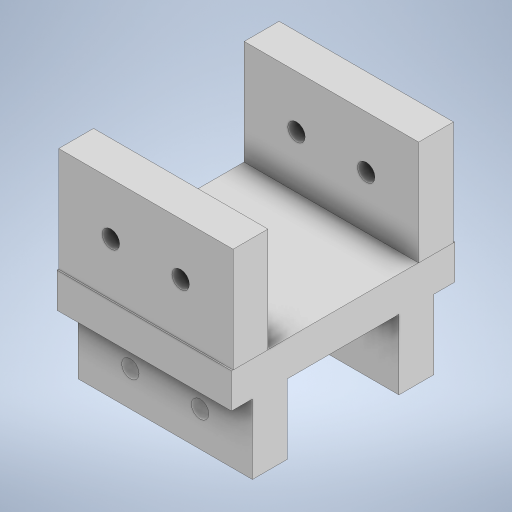
# Autodesk Inventor part: Tensile_test_bottom_adapter2
Saved by Autodesk Inventor 2024 (Build 280153000, 153)
## iProperties
Created: 2023-10-26
Part Number: Tensile_test_bottom_adapter2
Material: 일반
Document SubType Name: Modeling
Designer: jsw
Density: 1 g/cm^3
Appearance: 기본값
Author: jsw
Autodesk Inventor part; units mm, degrees
ref_plane "YZ Plane" through (0, 0, 0) normal (1, 0, 0) x (0, 1, 0)
ref_plane "XZ Plane" through (0, 0, 0) normal (0, 1, 0) x (-1, 0, 0)
ref_plane "XY Plane" through (0, 0, 0) normal (0, 0, 1) x (1, 0, 0)
sketch "스케치1" plane through (0, 0, 0) normal (0, 1, 0) x (-1, 0, 0)
  line L0 (-12.5, 16) -> (12.5, 16)
  line L1 (12.5, 16) -> (12.5, -16)
  line L2 (12.5, -16) -> (-12.5, -16)
  line L3 (-12.5, -16) -> (-12.5, 16)
  line L4 (-12.5, 16) -> (12.5, -16) construction
  line L5 (12.5, 16) -> (-12.5, -16) construction
  point P0 (0, 0)
  dimension "d0" = 25
  dimension "d1" = 32
  constraints: 12 end point, 2 midpoint, 2 parallel, 1 horizontal, 1 perpendicular
  measures "d0" distance of L1.end L2.end
  measures "d1" distance of L0.end L1.end
extrude "돌출1" add sketch "스케치1" along normal blind 5
sketch "스케치2" plane through (0, 5, 0) normal (0, 1, 0) x (1, 0, 0)
  line L0 (-12.4719, -15.8) -> (12.5281, -15.8)
  line L1 (12.5281, -15.8) -> (12.5281, -10.8)
  line L2 (12.5281, -10.8) -> (-12.4719, -10.8)
  line L3 (-12.4719, -10.8) -> (-12.4719, -15.8)
  line L4 (-12.5, 16) -> (-12.5, -16) projected
  line L5 (-12.5, 0) -> (12.5281, 0)
  line L6 (-12.4719, 15.8) -> (12.5281, 15.8)
  line L7 (12.5281, 15.8) -> (12.5281, 10.8)
  line L8 (12.5281, 10.8) -> (-12.4719, 10.8)
  line L9 (-12.4719, 10.8) -> (-12.4719, 15.8)
  line L10 (-12.5, -16) -> (-12.5, 16)
  point P0 (0, 0)
  dimension "d4" = 25
  dimension "d5" = 5
  dimension "d24" = 21.6
  constraints: 20 end point, 6 symmetric about line, 2 horizontal, 2 parallel, 1 midpoint, 1 perpendicular
  measures "d4" distance of L2.end L1.end
  measures "d5" distance of L1.end L0.end
  measures "d24" distance between parallel lines of L8 L2
extrude "돌출2" add sketch "스케치2" along normal blind 15
sketch "스케치3" plane through (12.5, 5, -15.8) normal (0, 0, -1) x (-1, 0, 0)
  circle A0 centre (7.4824, 7.5) radius 1.25
  line L0 (12.5, -5) -> (12.4719, 15)
  line L1 (24.9719, 15) -> (-0.0281, 15) projected
  line L2 (0, 0) -> (25, 0) projected
  circle A1 centre (17.4824, 7.514) radius 1.25
  dimension "d8" = 2.5
  dimension "d9" = 5
  dimension "d10" = 7.5
  constraints: 2 centre point, 2 end point, 1 midpoint, 1 symmetric about line, 1 other
  measures "d8" diameter of A0
  measures "d9" distance from line of L0 A0.centre
  measures "d10" distance from line of A0.centre L2
extrude "돌출3" cut sketch "스케치3" against normal up to surface (31.6 mm away)
sketch "스케치4" plane through (0, 0, 0) normal (0, -1, 0) x (1, 0, 0)
  line L0 (-12.5, -16) -> (-12.5, 16) projected
  line L1 (12.5, 10.8) -> (12.5, -10.8) projected
  line L2 (-12.5, 13) -> (12.5, 13)
  line L3 (12.5, 13) -> (12.5, 8)
  line L4 (12.5, 8) -> (-12.5, 8)
  line L5 (-12.5, 8) -> (-12.5, 13)
  line L6 (-12.5, 0) -> (12.5, 0)
  line L7 (-12.5, 16) -> (-12.5, -16)
  line L8 (12.5, -10.8) -> (12.5, 10.8)
  line L9 (-12.5, -13) -> (12.5, -13)
  line L10 (12.5, -13) -> (12.5, -8)
  line L11 (12.5, -8) -> (-12.5, -8)
  line L12 (-12.5, -8) -> (-12.5, -13)
  point P0 (0, 0)
  point P1 (12.5, -8)
  point P2 (-12.5, -13)
  dimension "d13" = 8
  dimension "d14" = 5
  constraints: 22 end point, 8 symmetric about line, 4 point on line, 2 midpoint, 2 parallel, 1 horizontal, 1 perpendicular
  measures "d13" distance from line of point (0, 0) L4
  measures "d14" distance of L2.end L3.end
extrude "돌출4" add sketch "스케치4" along normal blind 10 contours L0 L11 L1 L10 L9 | L0 L2 L3 L1 L4
sketch "스케치5" plane through (12.5, 0, -13) normal (0, 0, -1) x (-1, 0, 0)
  circle A0 centre (17.5, -5) radius 1.25
  line L0 (25, -10) -> (0, -10) projected
  line L1 (25, 0) -> (25, -10) projected
  line L2 (12.5, -10) -> (12.5, 0)
  circle A1 centre (7.5, -5) radius 1.25
  dimension "d17" = 2.5
  dimension "d18" = 5
  dimension "d22" = 5
  constraints: 2 centre point, 2 end point, 1 midpoint, 1 symmetric about line, 1 vertical, 1 other
  measures "d17" diameter of A0
  measures "d18" distance from line of A0.centre L0
  measures "d22" distance from line of L2 A0.centre
extrude "돌출5" cut sketch "스케치5" against normal up to surface (26 mm away)
